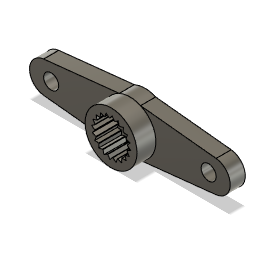
servo_horn_j3 (Autodesk Fusion 360 design; units mm, degrees)
Autodesk Fusion 360 part; units mm, degrees
sketch "Sketch1" plane through (0, 0, 2.25004) normal (0, 0, 1) x (1, 0, 0)
  line L0 (-1.997973, 1.636872) -> (-1.861856, 1.123701)
  line L1 (-1.997973, 1.636872) -> (-1.471475, 1.601775)
  line L2 (-1.471475, 1.601775) -> (-1.423653, 1.644443)
  line L3 (-1.423653, 1.644443) -> (-1.394411, 2.174404)
  line L4 (-1.394411, 2.174404) -> (-0.904354, 1.977965)
  line L5 (-0.904354, 1.977965) -> (-0.846392, 2.003911)
  line L6 (-0.846392, 2.003911) -> (-0.654777, 2.498375)
  line L7 (-0.654777, 2.498375) -> (-0.248384, 2.161444)
  line L8 (-0.248384, 2.161444) -> (-0.18548, 2.167944)
  line L9 (-0.18548, 2.167944) -> (0.149612, 2.578558)
  line L10 (0.149612, 2.578558) -> (0.430778, 2.132767)
  line L11 (0.430778, 2.132767) -> (0.493539, 2.119095)
  line L12 (0.493539, 2.119095) -> (0.93859, 2.406417)
  line L13 (0.93859, 2.406417) -> (1.068732, 1.894595)
  line L14 (1.068732, 1.894595) -> (1.124371, 1.862165)
  line L15 (1.124371, 1.862165) -> (1.636441, 1.998374)
  line L16 (1.601339, 1.471775) -> (1.636441, 1.998374)
  line L17 (1.601339, 1.471775) -> (1.643996, 1.423943)
  line L18 (1.643996, 1.423943) -> (2.173854, 1.394711)
  line L19 (1.978447, 0.904496) -> (2.173854, 1.394711)
  line L20 (1.978447, 0.904496) -> (2.003382, 0.846581)
  line L21 (2.003382, 0.846581) -> (2.498752, 0.654883)
  line L22 (2.160873, 0.24846) -> (2.498752, 0.654883)
  line L23 (2.160873, 0.24846) -> (2.167368, 0.185545)
  line L24 (2.167368, 0.185545) -> (2.578902, -0.149663)
  line L25 (2.132185, -0.430832) -> (2.578902, -0.149663)
  line L26 (2.118515, -0.493605) -> (2.132185, -0.430832)
  line L27 (2.118515, -0.493605) -> (2.406776, -0.938797)
  line L28 (1.894045, -1.068915) -> (2.406776, -0.938797)
  line L29 (1.862682, -1.123617) -> (1.894045, -1.068915)
  line L30 (1.862682, -1.123617) -> (1.997793, -1.636734)
  line L31 (1.471295, -1.601637) -> (1.997793, -1.636734)
  line L32 (1.423473, -1.644301) -> (1.471295, -1.601637)
  line L33 (1.394232, -2.174263) -> (1.423473, -1.644301)
  line L34 (0.90518, -1.97788) -> (1.394232, -2.174263)
  line L35 (0.846213, -2.003768) -> (0.90518, -1.97788)
  line L36 (0.654597, -2.498233) -> (0.846213, -2.003768)
  line L37 (0.249209, -2.161364) -> (0.654597, -2.498233)
  line L38 (0.185301, -2.167802) -> (0.249209, -2.161364)
  line L39 (-0.149849, -2.579426) -> (0.185301, -2.167802)
  line L40 (-0.430957, -2.132626) -> (-0.149849, -2.579426)
  line L41 (-0.492713, -2.119015) -> (-0.430957, -2.132626)
  line L42 (-0.938827, -2.40728) -> (-0.492713, -2.119015)
  line L43 (-1.068912, -1.894453) -> (-0.938827, -2.40728)
  line L44 (-1.123545, -1.86208) -> (-1.068912, -1.894453)
  line L45 (-1.636621, -1.998236) -> (-1.123545, -1.86208)
  line L46 (-1.636621, -1.998236) -> (-1.601519, -1.471634)
  line L47 (-1.644175, -1.423805) -> (-1.601519, -1.471634)
  line L48 (-2.174034, -1.394569) -> (-1.644175, -1.423805)
  line L49 (-2.174034, -1.394569) -> (-1.977621, -0.904412)
  line L50 (-2.003561, -0.846439) -> (-1.977621, -0.904412)
  line L51 (-2.498931, -0.654741) -> (-2.003561, -0.846439)
  line L52 (-2.498931, -0.654741) -> (-2.16111, -0.249324)
  line L53 (-2.167547, -0.185403) -> (-2.16111, -0.249324)
  line L54 (-2.579081, 0.149801) -> (-2.167547, -0.185403)
  line L55 (-2.579081, 0.149801) -> (-2.132364, 0.430974)
  line L56 (-2.132364, 0.430974) -> (-2.118753, 0.492742)
  line L57 (-2.406955, 0.938935) -> (-2.118753, 0.492742)
  line L58 (-2.406955, 0.938935) -> (-1.894224, 1.069057)
  line L59 (-1.894224, 1.069057) -> (-1.861856, 1.123701)
  circle A0 centre (0, 0) radius 3.45
  point P0 (0.106248, 3.448364)
  constraint coincident A0.centre origin
surface "SurfacePatch1" add patch profiles "Sketch1" section 1 contours A0 picked at (-1.433482, -2.464435) makes body 1
extrude "Extrude1" add 1 faces at (-1.433482, -2.464435, 2.25004) along direction (0, 0, -1) blind 3 separate body on bodies 1 makes body 2
sketch "Sketch2" plane through (-0.000001, 0, -2.250037) normal (0, 0, -1) x (-1, 0, 0)
  circle A0 centre (0, 0) radius 2.625
  circle A1 centre (-10.450008, 0.000012) radius 1
  circle A2 centre (10.449992, 0.000012) radius 1
  line L0 (1.410863, 3.148325) -> (11.441192, 2.080174)
  line L1 (1.40705, -3.15003) -> (11.439375, -2.096922)
  arc A3 (11.439375, -2.096922) -> (11.441192, 2.080174) centre (11.220127, -0.008278) ccw
  line L2 (-11.439374, 2.096899) -> (-1.410863, 3.148325)
  line L3 (-11.441193, -2.080199) -> (-1.407052, -3.15003)
  arc A4 (-11.439374, 2.096899) -> (-11.441193, -2.080199) centre (-11.218524, 0.008254) ccw
  arc A5 (1.410863, 3.148325) -> (-1.410863, 3.148325) centre (0, 0) ccw
  arc A6 (-1.407052, -3.15003) -> (1.40705, -3.150031) centre (0, 0) ccw
  point P0 (-11.439374, 2.096899)
  point P1 (-11.441193, -2.080199)
  point P2 (9.449992, 0.000011)
  point P3 (11.449992, 0.000012)
  point P4 (11.441192, 2.080174)
  point P5 (11.439375, -2.096922)
  point P6 (-11.450008, 0.000011)
  point P7 (-9.450008, 0.000012)
  constraint coincident A0.centre A5.centre
  constraint tangent L1 A3
  constraint tangent L3 A4
  constraint concentric A5 A6
surface "SurfacePatch2" add patch profiles "Sketch2" section 1 contours L0 L1 A3 L2 L3 A4 A5 A6 picked at (7.598806, -2.037656) separate body makes body 3
extrude "Extrude2" add 1 faces at (-7.598806, -2.037656, -2.250035) along direction (0.00000026, 0.00000003, 1) blind 2 separate body on bodies 3 makes body 4
sketch "Sketch3" plane through (0, 0, -1.250038) normal (0, 0, -1) x (-1, 0, 0)
  circle A0 centre (0, 0) radius 1.299989
  circle A1 centre (0, 0) radius 2.701851
  point P0 (-0.032415, 1.299585)
  constraint coincident A0.centre A1.centre
surface "SurfacePatch3" add patch profiles "Sketch3" section 1 contours A1 picked at (2.219665, -0.198814) separate body makes body 5
extrude "Extrude3" add 1 faces at (-2.219665, -0.198814, -1.250038) along direction (0, 0, 1) blind 0.5 separate body on bodies 5 makes body 6
combine "Combine1" operation add target body 4 tool bodies 2 6
hidden bodies 1 3 5
